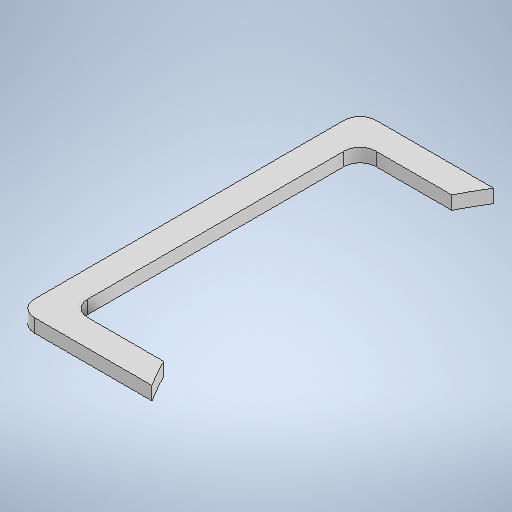
# Autodesk Inventor part: handlebar
Saved by Autodesk Inventor 2025.2 (Build 292293000, 293)
## iProperties
Created: 2025-06-08
Part Number: handlebar
Material: Generic
Document SubType Name: Modeling
Designer: gasla
Density: 1 g/cm^3
Appearance: Default
Author: gasla
Autodesk Inventor part; units mm, degrees
ref_plane "YZ Plane" through (0, 0, 0) normal (1, 0, 0) x (0, 1, 0)
ref_plane "XZ Plane" through (0, 0, 0) normal (0, 1, 0) x (-1, 0, 0)
ref_plane "XY Plane" through (0, 0, 0) normal (0, 0, 1) x (1, 0, 0)
sketch "Sketch1" plane through (0, 0, 0) normal (0, 1, 0) x (-1, 0, 0)
  circle A0 centre (0, 0) radius 600
  line L0 (0, 0) -> (507.7952, 0) construction
  line L1 (507.7952, 0) -> (507.7952, -319.5997) construction
  line L2 (507.7952, 0) -> (507.7952, 319.5997) construction
  line L3 (507.7952, 319.5997) -> (507.7952, 269.5997)
  line L4 (507.7952, -319.5997) -> (507.7952, -269.5997)
  line L5 (507.7952, 319.5997) -> (727.7952, 319.5997)
  line L6 (507.7952, -319.5997) -> (727.7952, -319.5997)
  line L7 (757.7952, -289.5997) -> (757.7952, 289.5997)
  line L8 (707.7952, 239.5997) -> (707.7952, -239.5997)
  line L9 (507.7952, -269.5997) -> (677.7952, -269.5997)
  line L10 (507.7952, 269.5997) -> (677.7952, 269.5997)
  arc A1 (757.7952, 289.5997) -> (727.7952, 319.5997) centre (727.7952, 289.5997) ccw
  arc A2 (727.7952, -319.5997) -> (757.7952, -289.5997) centre (727.7952, -289.5997) ccw
  arc A3 (677.7952, -269.5997) -> (707.7952, -239.5997) centre (677.7952, -239.5997) ccw
  arc A4 (707.7952, 239.5997) -> (677.7952, 269.5997) centre (677.7952, 239.5997) ccw
  point P0 (757.7952, 319.5997)
  point P1 (707.7952, 319.5997)
  point P2 (707.7952, -319.5997)
  point P3 (536.0186, 269.5997)
  point P4 (536.0186, -269.5997)
  dimension "d0" = 1200
  dimension "d1" = 50
  dimension "d2" = 319.5997
  dimension "d3" = 50
  dimension "d4" = 250
  dimension "d7" = 50
  dimension "d8" = 30
  dimension "d9" = 30
  dimension "d10" = 30
  dimension "d11" = 30
  constraints: 22 end point, 10 point on circle, 8 point on line, 8 tangent, 5 centre point, 3 horizontal, 3 perpendicular, 2 vertical, 1 coincident
  measures "d0" diameter of A0
  measures "d1" distance of L2.end L3.end
  measures "d2" distance of L0.end L2.end
  measures "d3" distance of L4.end L1.end
  measures "d4" distance of L2.end point (757.795, 319.6)
  measures "d7" distance between parallel lines of L7 L8
  measures "d8" radius of A1
  measures "d9" radius of A2
  measures "d10" radius of A3
  measures "d11" radius of A4
extrude "Extrusion1" add sketch "Sketch1" along normal blind 25 contours L5 A1 L7 A2 L6 A0 L9 A3 L8 A4 L10
body "Solid1"
